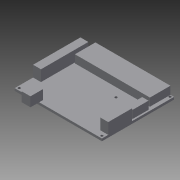
# Autodesk Inventor part: Megatronics3.0
Saved by Autodesk Inventor 2015 (Build 190159000, 159)
## iProperties
Created: 2014-08-16
Part Number: Megatronics3.0
Material: Generic
Document SubType Name: Modeling
Designer: Jack
Density: 1 g/cm^3
Appearance: Default
Author: Jack
Autodesk Inventor part; units mm, degrees
ref_plane "YZ Plane" through (0, 0, 0) normal (1, 0, 0) x (0, 1, 0)
ref_plane "XZ Plane" through (0, 0, 0) normal (0, 1, 0) x (-1, 0, 0)
ref_plane "XY Plane" through (0, 0, 0) normal (0, 0, 1) x (1, 0, 0)
sketch "Sketch1" plane through (0, 0, 0) normal (0, 0, 1) x (1, 0, 0)
  line L0 (0, 0) -> (110.5, 0)
  line L1 (110.5, 0) -> (110.5, 91.3)
  line L2 (110.5, 91.3) -> (0, 91.3)
  line L3 (0, 91.3) -> (0, 0)
  circle A0 centre (2.8, 3) radius 1.5
  circle A1 centre (74.3, 54.1) radius 1.5
  circle A2 centre (3.6, 88.5) radius 1.5
  circle A3 centre (107.5, 3) radius 1.5
  circle A4 centre (107.8, 89) radius 1.5
  dimension "d0" = 110.5
  dimension "d1" = 91.3
  dimension "d2" = 3
  dimension "d3" = 3
  dimension "d4" = 3
  dimension "d5" = 3
  dimension "d6" = 3
  dimension "d7" = 2.8
  dimension "d8" = 3
  dimension "d9" = 3.6
  dimension "d10" = 88.5
  dimension "d11" = 74.3
  dimension "d12" = 54.1
  dimension "d13" = 107.5
  dimension "d14" = 3
  dimension "d15" = 89
  dimension "d16" = 107.8
  constraints: 8 end point, 5 centre point, 2 parallel, 1 horizontal, 1 perpendicular
  measures "d0" distance of L2.end L1.end
  measures "d1" distance of L1.end L0.end
  measures "d2" diameter of A0
  measures "d3" diameter of A1
  measures "d4" diameter of A2
  measures "d5" diameter of A3
  measures "d6" diameter of A4
  measures "d7" distance from line of L3 A0.centre
  measures "d8" distance from line of L0 A0.centre
  measures "d9" distance from line of L3 A2.centre
  measures "d10" distance from line of L0 A2.centre
  measures "d11" distance from line of L3 A1.centre
  measures "d12" distance from line of L0 A1.centre
  measures "d13" distance from line of L3 A3.centre
  measures "d14" distance from line of L0 A3.centre
  measures "d15" distance from line of L0 A4.centre
  measures "d16" distance from line of L3 A4.centre
extrude "Extrusion1" add sketch "Sketch1" along normal blind 3
sketch "Sketch2" plane through (0, 0, 3) normal (0, 0, 1) x (1, 0, 0)
  line L0 (110.5, 91.3) -> (0, 91.3) projected
  line L1 (0, 91.3) -> (0, 0) projected
  line L2 (0, 83.3) -> (10, 83.3)
  line L3 (10, 83.3) -> (10, 23.3)
  line L4 (10, 23.3) -> (0, 23.3)
  line L5 (0, 23.3) -> (0, 83.3)
  dimension "d19" = 10
  dimension "d20" = 60
  dimension "d21" = 8
  constraints: 8 end point, 2 parallel, 1 horizontal, 1 perpendicular, 1 point on line
  measures "d19" distance of L3.end L4.end
  measures "d20" distance of L2.end L3.end
  measures "d21" distance between parallel lines of L0 L2
extrude "Extrusion2" add sketch "Sketch2" along normal blind 14
sketch "Sketch3" plane through (0, 0, 3) normal (0, 0, 1) x (1, 0, 0)
  line L0 (110.5, 0) -> (110.5, 91.3) projected
  line L1 (110.5, 91.3) -> (0, 91.3) projected
  line L2 (106, 91.3) -> (11, 91.3)
  line L3 (11, 91.3) -> (11, 65.3)
  line L4 (11, 65.3) -> (106, 65.3)
  line L5 (106, 65.3) -> (106, 91.3)
  dimension "d24" = 95
  dimension "d25" = 26
  dimension "d26" = 0
  dimension "d27" = 4.5
  constraints: 8 end point, 2 parallel, 1 horizontal, 1 perpendicular
  measures "d24" distance of L4.end L3.end
  measures "d25" distance of L3.end L2.end
  measures "d26" distance between parallel lines of L1 L2
  measures "d27" distance between parallel lines of L0 L5
extrude "Extrusion3" add sketch "Sketch3" along normal blind 10
sketch "Sketch4" plane through (0, 0, 3) normal (0, 0, 1) x (1, 0, 0)
  line L0 (0, 23.3) -> (0, 0) projected
  line L1 (0, 0) -> (110.5, 0) projected
  line L2 (20, 5) -> (31, 5)
  line L3 (31, 5) -> (31, -11)
  line L4 (31, -11) -> (20, -11)
  line L5 (20, -11) -> (20, 5)
  dimension "d30" = 11
  dimension "d31" = 16
  dimension "d32" = 20
  dimension "d33" = 5
  constraints: 8 end point, 2 parallel, 1 horizontal, 1 perpendicular
  measures "d30" distance of L2.start L2.end
  measures "d31" distance of L4.end L2.start
  measures "d32" distance between parallel lines of L0 L5
  measures "d33" distance between parallel lines of L1 L2
extrude "Extrusion4" add sketch "Sketch4" along normal blind 12
sketch "Sketch5" plane through (0, 0, 3) normal (0, 0, 1) x (1, 0, 0)
  line L0 (31, 0) -> (110.5, 0) projected
  line L1 (110.5, 0) -> (110.5, 91.3) projected
  line L2 (110.5, 8) -> (100.5, 8)
  line L3 (100.5, 8) -> (100.5, 38)
  line L4 (100.5, 38) -> (110.5, 38)
  line L5 (110.5, 38) -> (110.5, 8)
  dimension "d36" = 10
  dimension "d37" = 30
  dimension "d38" = 8
  constraints: 8 end point, 2 parallel, 1 horizontal, 1 perpendicular, 1 point on line
  measures "d36" distance of L3.end L4.end
  measures "d37" distance of L2.end L3.end
  measures "d38" distance between parallel lines of L0 L2
extrude "Extrusion5" add sketch "Sketch5" along normal blind 14
sketch "Sketch6" plane through (0, 0, 3) normal (0, 0, 1) x (1, 0, 0)
  line L0 (100.5, 38) -> (110.5, 38) projected
  line L1 (110.5, 38) -> (110.5, 91.3) projected
  line L2 (100.5, 41) -> (108.5, 41)
  line L3 (108.5, 41) -> (108.5, 61)
  line L4 (108.5, 61) -> (100.5, 61)
  line L5 (100.5, 61) -> (100.5, 41)
  dimension "d41" = 8
  dimension "d42" = 2
  dimension "d43" = 3
  dimension "d44" = 20
  constraints: 8 end point, 2 parallel, 1 horizontal, 1 perpendicular
  measures "d41" distance of L4.end L3.end
  measures "d42" distance between parallel lines of L1 L3
  measures "d43" distance between parallel lines of L0 L2
  measures "d44" distance of L4.end L2.start
extrude "Extrusion6" add sketch "Sketch6" along normal blind 10
body "Solid1"
